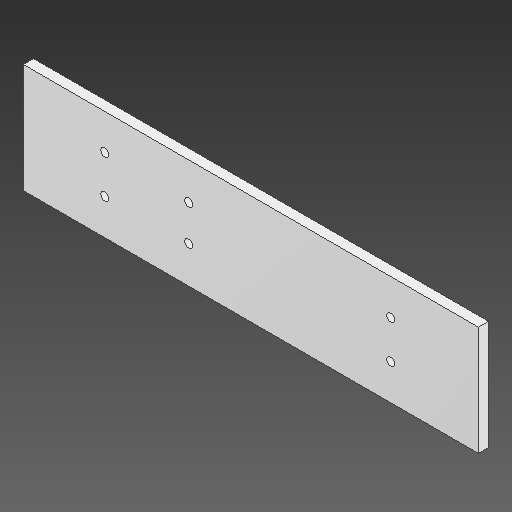
# Autodesk Inventor part: FrontWallUHMW
Saved by Autodesk Inventor 2021 (Build 250183000, 183)
## iProperties
Created: 2021-03-10
Part Number: FrontWallUHMW
Material: UHMW, White
Document SubType Name: Modeling
Designer: Dylan
Density: 0.94 g/cm^3
Appearance: Smooth - White
Mass: 920.556 g
Surface Area: 1745.4 cm^2
Volume: 979.315 cm^3
Author: Dylan
Autodesk Inventor part; units mm, degrees
ref_plane "YZ Plane" through (0, 0, 0) normal (1, 0, 0) x (0, 1, 0)
ref_plane "XZ Plane" through (0, 0, 0) normal (0, 1, 0) x (-1, 0, 0)
ref_plane "XY Plane" through (0, 0, 0) normal (0, 0, 1) x (1, 0, 0)
sketch "Sketch1" plane through (0, 0, 0) normal (0, 0, 1) x (1, 0, 0)
  line L0 (0, -3.175) -> (568.325, -3.175)
  line L1 (568.325, -3.175) -> (568.325, 133.35)
  line L2 (568.325, 133.35) -> (0, 133.35)
  line L3 (0, 133.35) -> (0, -3.175)
  line L4 (1244.6, -3.175) -> (25.4, -3.175) projected
  line L5 (568.325, 115.8875) -> (568.325, 14.2875) projected
  line L6 (0, 71.4375) -> (0, 103.1875)
  line L7 (539.75, 133.35) -> (-679.45, 133.35)
  point P0 (539.75, -3.175)
  constraints: 12 end point, 4 point on line, 2 horizontal, 2 parallel, 1 perpendicular, 1 vertical, 5 other
extrude "Extrusion1" add sketch "Sketch1" along normal blind 12.7
sketch "Sketch2" plane through (0, 0, 12.7) normal (0, 0, 1) x (1, 0, 0)
  circle A0 centre (458.7875, 41.275) radius 5.0419
  circle A1 centre (458.7875, 88.9) radius 5.0419
  ellipse E0 centre (361.95, 39.714) end of major axis (358.6836, 39.714) minor radius 3.2664
  circle A2 centre (352.425, 87.3125) radius 5.0419
  circle A3 centre (352.425, 42.8625) radius 5.0419
  circle A4 centre (206.375, 42.8625) radius 5.0419
  circle A5 centre (206.375, 87.3125) radius 5.0419
  circle A6 centre (101.6, 88.9) radius 5.0419
  circle A7 centre (101.6, 41.275) radius 5.0419
  point P0 (0, 0)
  point P1 (99.2809, 89.5337)
  constraints: 8 centre point, 19 other
hole "Hole1" at (458.7875, 41.275, 12.7) at (458.7875, 88.9, 12.7) at (206.375, 42.8625, 12.7) at (206.375, 87.3125, 12.7) at (101.6, 41.275, 12.7) at (101.6, 88.9, 12.7) direction (0, 0, -1) diameter 10.0838 end through all clearance for "Hex Head Bolt" size "3/8" standard "Ansi Unified Screw Threads"
body "Solid1"
